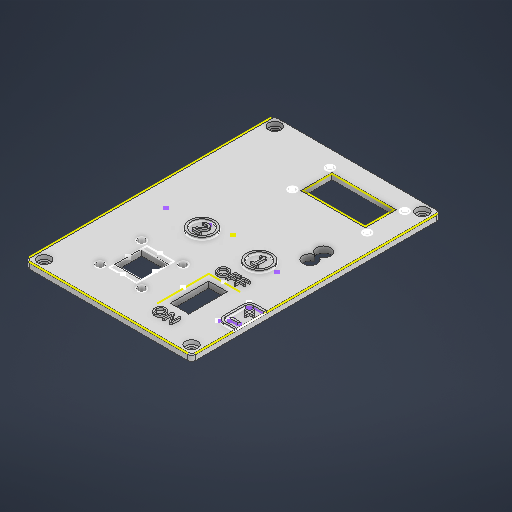
# Autodesk Inventor part: PCB_Housing_06_V4
Saved by Autodesk Inventor 2026.2 (Build 302298010, 298A)
## iProperties
Created: 2026-03-17
Part Number: PCB_Housing_06_V4
Material: Generic
Document SubType Name: Modeling
Designer: vckot
Density: 1 g/cm^3
Appearance: Default
Author: vckot
Autodesk Inventor part; units mm, degrees
ref_plane "YZ Plane" through (0, 0, 0) normal (1, 0, 0) x (0, 1, 0)
ref_plane "XZ Plane" through (0, 0, 0) normal (0, 1, 0) x (-1, 0, 0)
ref_plane "XY Plane" through (0, 0, 0) normal (0, 0, 1) x (1, 0, 0)
sketch "Sketch1" plane through (0, 0, 0) normal (0, 1, 0) x (-1, 0, 0)
  line L0 (-40, 60) -> (40, 60)
  line L1 (40, 60) -> (40, -60)
  line L2 (40, -60) -> (-40, -60)
  line L3 (-40, -60) -> (-40, 60)
  line L4 (-40, 60) -> (40, -60) construction
  line L5 (40, 60) -> (-40, -60) construction
  point P0 (0, 0)
  dimension "d0" = 120
  dimension "d1" = 80
  constraints: 12 end point, 2 midpoint, 2 parallel, 1 horizontal, 1 perpendicular
  measures "d0" distance of L0.end L1.end
  measures "d1" distance of L0.start L0.end
extrude "Extrusion1" add sketch "Sketch1" along normal blind 3
sketch "Sketch2" plane through (0, 3, 0) normal (0, 1, 0) x (1, 0, 0)
  circle A0 centre (35.5, 55.5) radius 2.25
  circle A1 centre (-35.5, -55.5) radius 2.25
  arc A2 (37.5, -54.469224) -> (34.469224, -57.5) centre (35.5, -55.5) ccw
  circle A3 centre (-35.5, 55.5) radius 2.25
  circle A4 centre (35.5, -55.5) radius 2.25
  point P0 (0, 0)
  constraints: 2 centre point, 2 horizontal alignment, 2 vertical alignment
hole "Hole1" at (35.5, 3, -55.5) at (-35.5, 3, 55.5) at (35.5, 3, 55.5) at (-35.5, 3, -55.5) direction (0, -1, 0) diameter 3.75 depth 8 tip angle 118 counterbore diameter 6 counterbore depth 2
sketch "Sketch3" plane through (0, 3, 0) normal (0, 1, 0) x (1, 0, 0)
  line L0 (24.241, -45.543499) -> (24.241, -22.556499)
  line L1 (10.779, -45.543499) -> (24.241, -45.543499)
  line L2 (10.779, -22.556499) -> (10.779, -45.543499)
  line L3 (10.779, -22.556499) -> (24.241, -22.556499)
  arc A0 (26.856832, 17.449996) -> (30.143167, 17.449996) centre (28.499999, 14.999996) ccw
  arc A1 (26.856832, 10.949996) -> (30.143167, 10.949996) centre (28.499999, 8.499996) ccw
  circle A2 centre (28.499999, 8.499996) radius 2.95
  circle A3 centre (28.499999, 14.999996) radius 2.95
  line L4 (28, 35.5) -> (-2, 35.5)
  line L5 (-2, 35.5) -> (-2, 49.5)
  line L6 (-2, 49.5) -> (28, 49.5)
  line L7 (28, 49.5) -> (28, 35.5)
  circle A4 centre (-7, 34) radius 1.1
  circle A5 centre (30, 34) radius 1.1
  circle A6 centre (30, 52) radius 1.1
  circle A7 centre (-7, 52) radius 1.1
  line L8 (31.5, 32.5) -> (31.5, 53.5)
  line L9 (31.5, 53.5) -> (-8.5, 53.5)
  line L10 (-8.5, 53.5) -> (-8.5, 32.5)
  line L11 (-8.5, 32.5) -> (31.5, 32.5)
  line L12 (24.241, -22.556499) -> (10.779, -22.556499)
  line L13 (10.779, -22.556499) -> (10.779, -45.543499)
  line L14 (10.779, -45.543499) -> (24.241, -45.543499)
  line L15 (24.241, -45.543499) -> (24.241, -22.556499)
  arc A8 (12.1379, -23.305799) -> (11.7569, -23.686799) centre (12.1379, -23.686799) ccw
  line L16 (11.7569, -23.686799) -> (11.7569, -23.153399)
  line L17 (11.7569, -23.153399) -> (23.2631, -23.153399)
  line L18 (23.2631, -23.153399) -> (23.2631, -23.686799)
  arc A9 (23.2631, -23.686799) -> (22.8821, -23.305799) centre (22.8821, -23.686799) ccw
  line L19 (22.8821, -23.305799) -> (20.05, -23.305799)
  line L20 (20.05, -23.305799) -> (20.05, -23.559799)
  line L21 (20.05, -23.559799) -> (14.97, -23.559799)
  line L22 (14.97, -23.559799) -> (14.97, -23.305799)
  line L23 (14.97, -23.305799) -> (12.1379, -23.305799)
  line L24 (18.790769, -42.147052) -> (18.797824, -42.147052)
  line L25 (18.797824, -42.147052) -> (19.407999, -41.186537)
  line L26 (19.407999, -41.186537) -> (20.174294, -41.186537)
  line L27 (20.174294, -41.186537) -> (19.317111, -42.295346)
  line L28 (19.317111, -42.295346) -> (19.71607, -43.707864)
  line L29 (19.71607, -43.707864) -> (18.921553, -43.707864)
  line L30 (18.921553, -43.707864) -> (18.739263, -42.870885)
  line L31 (18.739263, -42.870885) -> (18.595587, -43.065169)
  line L32 (18.595587, -43.065169) -> (18.458966, -43.707864)
  line L33 (18.458966, -43.707864) -> (17.828648, -43.707864)
  line L34 (17.828648, -43.707735) -> (17.358303, -43.707735)
  line L35 (17.358303, -43.707735) -> (17.312378, -43.618194)
  spline S0 degree 3 poles (17.312378, -43.618194) (17.183262, -43.69882) (17.011235, -43.7391) (16.883594, -43.7391) knots 0 0 0 0 1 1 1 1
  spline S1 degree 3 poles (16.883594, -43.7391) (16.666279, -43.7391) (16.455181, -43.56555) (16.493385, -43.215144) (16.643637, -42.986824) (16.809283, -42.872511) (16.900399, -42.827654) knots 0.00500991 0.00500991 0.00500991 0.00500991 0.25104614 0.49708236 0.74311859 0.98915482 0.98915482 0.98915482 0.98915482
  spline S2 degree 3 poles (16.900399, -42.827654) (16.834462, -42.726888) (16.785779, -42.608163) (16.814322, -42.473787) knots 0 0 0 0 1 1 1 1
  spline S3 degree 3 poles (16.814322, -42.473787) (16.865314, -42.234156) (17.088333, -42.0908) (17.343615, -42.0908) knots 0 0 0 0 1 1 1 1
  spline S4 degree 3 poles (17.343615, -42.0908) (17.467218, -42.0908) (17.681137, -42.129323) (17.798163, -42.294936) (17.752062, -42.538795) (17.638072, -42.718098) (17.498782, -42.813553) (17.399546, -42.881404) knots 0.00821535 0.00821535 0.00821535 0.00821535 0.2540357 0.49985605 0.62276622 0.74567639 0.99149674 0.99149674 0.99149674 0.99149674
  line L36 (17.399546, -42.881404) -> (17.51019, -43.09865)
  spline S5 degree 3 poles (17.51019, -43.09865) (17.548931, -43.042655) (17.587672, -42.98666) (17.601014, -42.92393) knots 0 0 0 0 1 1 1 1
  line L37 (17.601014, -42.92393) -> (17.91933, -42.92393)
  line L38 (17.91933, -42.92393) -> (18.288607, -41.186537)
  line L39 (18.288607, -41.186537) -> (18.994866, -41.186537)
  line L40 (18.994866, -41.186537) -> (18.790769, -42.147052)
  line L41 (16.779109, -42.103629) -> (16.094081, -42.103629)
  line L42 (16.094081, -42.103629) -> (16.137569, -41.898762)
  spline S6 degree 3 poles (16.137569, -41.898762) (16.160852, -41.789337) (16.203698, -41.588062) (16.058867, -41.588062) knots 0 0 0 0 1 1 1 1
  spline S7 degree 3 poles (16.058867, -41.588062) (15.875231, -41.588062) (15.841172, -41.715125) (15.688773, -42.432031) knots 0 0 0 0 1 1 1 1
  spline S8 degree 3 poles (15.688773, -42.432031) (15.531947, -43.17004) (15.527073, -43.275937) (15.700062, -43.275937) knots 0 0 0 0 1 1 1 1
  spline S9 degree 3 poles (15.700062, -43.275937) (15.813078, -43.275937) (15.883056, -43.162984) (15.949827, -42.848693) knots 0 0 0 0 1 1 1 1
  line L43 (15.949827, -42.848693) -> (15.99107, -42.654473)
  line L44 (15.99107, -42.654473) -> (16.676162, -42.654473)
  line L45 (16.676162, -42.654473) -> (16.642424, -42.813415)
  spline S10 degree 3 poles (16.642424, -42.813415) (16.517028, -43.403065) (16.20838, -43.742115) (15.590444, -43.742115) knots 0.00895212 0.00895212 0.00895212 0.00895212 0.99175551 0.99175551 0.99175551 0.99175551
  spline S11 degree 3 poles (15.590444, -43.742115) (15.27401, -43.742115) (14.887863, -43.619986) (14.820678, -43.200507) (14.894815, -42.739756) (15.015532, -42.174372) (15.128196, -41.693261) (15.356087, -41.359939) (15.610614, -41.189827) (15.990864, -41.109001) (16.642583, -41.140034) (16.885652, -41.421424) (16.852223, -41.758005) (16.818145, -41.919923) knots 0.00651356 0.00651356 0.00651356 0.00651356 0.12992302 0.25333248 0.31503721 0.37674194 0.5001514 0.56185613 0.62356086 0.68526559 0.74697032 0.87037978 0.98786975 0.98786975 0.98786975 0.98786975
  line L46 (16.818171, -41.919928) -> (16.779109, -42.103629)
  line L47 (14.5255, -39.993599) -> (14.5255, -28.106399)
  line L48 (14.5255, -28.106399) -> (20.4945, -28.106399)
  line L49 (20.4945, -28.106399) -> (20.4945, -39.993599)
  line L50 (20.4945, -39.993599) -> (14.5255, -39.993599)
  arc A10 (22.8821, -44.794199) -> (23.2631, -44.413199) centre (22.8821, -44.413199) ccw
  line L51 (23.2631, -44.413199) -> (23.2631, -44.946599)
  line L52 (23.2631, -44.946599) -> (11.7569, -44.946599)
  line L53 (11.7569, -44.946599) -> (11.7569, -44.413199)
  arc A11 (11.7569, -44.413199) -> (12.1379, -44.794199) centre (12.1379, -44.413199) ccw
  line L54 (12.1379, -44.794199) -> (22.8821, -44.794199)
  point P0 (0, 0)
  point P1 (26.856832, 10.949996)
extrude "Extrusion2" cut sketch "Sketch3" against normal through all contours L1 L2 L3 L0 | A3 A0 | A2 A1 | L4 L5 L6 L7 | A8 L16 L17 L18 A9 L19 L20 L21 L22 L23 | L24 L25 L26 L27 L28 L29 L30 L31 L32 L33 L34 L35 S0 S1 S2 S3 S4 L36 S5 L37 L38 L39 L40 | L41 L42 S6 S7 S8 S9 L43 L44 L45 S10 S11 L46 | L47 L48 L49 L50 | A10 L51 L52 L53 A11 L54
sketch "Sketch5" plane through (0, 3, 0) normal (0, 1, 0) x (1, 0, 0)
  circle A0 centre (-5, 33.5) radius 1.75
  circle A1 centre (-5, 51.5) radius 1.75
  circle A2 centre (31, 51.5) radius 1.75
  circle A3 centre (31, 33.5) radius 1.75
  line L0 (28, 35.5) -> (-2, 35.5) projected
  line L1 (-2, 35.5) -> (-2, 49.5) projected
  line L2 (-2, 49.5) -> (28, 49.5) projected
  line L3 (28, 49.5) -> (28, 35.5) projected
  point P0 (0, 0)
  dimension "d27" = 3.5
  dimension "d28" = 2
  dimension "d29" = 3
  dimension "d30" = 2
  dimension "d31" = 3
  dimension "d32" = 3
  dimension "d33" = 3
  dimension "d34" = 2
  dimension "d35" = 2
  constraints: 4 centre point, 3 equal radius
  measures "d27" diameter of A0
  measures "d28" distance from line of A0.centre L0
  measures "d29" distance from line of L1 A0.centre
  measures "d30" distance from line of L2 A1.centre
  measures "d31" distance from line of L1 A1.centre
  measures "d32" distance from line of L3 A2.centre
  measures "d33" distance from line of L3 A3.centre
  measures "d34" distance from line of L0 A3.centre
  measures "d35" distance from line of L2 A2.centre
thicken "Thicken1" operation add thickness 0.5 both sides no extend neighbours yes toward (0, 0, -1) faces at (18, 2, -49.5) (-2, 2, -44.833333) (28, 2, -40.166667) (8, 2, -35.5)
thicken "Thicken2" operation add thickness 0.5 both sides no extend neighbours yes toward (0.6830158, 0, -0.7304036) faces at (30.514896, 2, -17.154687)
thicken "Thicken3" operation add thickness 0.5 both sides no extend neighbours yes toward (0.6830158, 0, -0.7304036) faces at (30.514896, 2, -10.654687)
thicken "Thicken4" operation add thickness 0.75 both sides no extend neighbours yes toward (1, 0, 0) faces at (24.241, 2, 37.881166) (15.266333, 1, 22.556499) (10.779, 2, 30.218832) (15.266333, 2, 45.543499)
sketch "Sketch4" plane through (0, 3, 0) normal (0, 1, 0) x (1, 0, 0)
  line L0 (7.168033, -20.561799) -> (27.698693, -20.561798) construction
  line L1 (27.698693, -20.561798) -> (27.698693, -47.5382) construction
  line L2 (27.698693, -47.5382) -> (7.168033, -47.5382) construction
  line L3 (7.168033, -47.5382) -> (7.168033, -20.561799) construction
  line L4 (10.029, -21.806499) -> (24.991, -21.806499)
  line L5 (10.029, -46.293499) -> (10.029, -21.806499)
  spline S0 degree 2 poles (13.32574, -20.740761) (12.567892, -20.740761) (11.464753, -20.090537) (10.854888, -18.94704) (10.841435, -18.207129) knots 0 0 0 1 2 3 3 3
  spline S1 degree 2 poles (10.841435, -18.207129) (10.854888, -17.467219) (11.460269, -16.323721) (12.567892, -15.673497) (13.32574, -15.673497) knots 0 0 0 1 2 3 3 3
  spline S2 degree 2 poles (13.32574, -15.673497) (14.079103, -15.673497) (15.182242, -16.323721) (15.792107, -17.467219) (15.80556, -18.207129) knots 0 0 0 1 2 3 3 3
  spline S3 degree 2 poles (15.80556, -18.207129) (15.792107, -18.947039) (15.182242, -20.090537) (14.079103, -20.740761) (13.32574, -20.740761) knots 0 0 0 1 2 3 3 3
  spline S4 degree 2 poles (13.32574, -20.018788) (13.872825, -20.018788) (14.635157, -19.538968) (15.038744, -18.71834) (15.038744, -18.207129) knots 0 0 0 1 2 3 3 3
  spline S5 degree 2 poles (15.038744, -18.207129) (15.038744, -17.695918) (14.635157, -16.875291) (13.872825, -16.39547) (13.32574, -16.39547) knots 0 0 0 1 2 3 3 3
  spline S6 degree 2 poles (13.32574, -16.39547) (12.77417, -16.39547) (12.011838, -16.875291) (11.612735, -17.691434) (11.612735, -18.207129) knots 0 0 0 1 2 3 3 3
  spline S7 degree 2 poles (11.612735, -18.207129) (11.612735, -18.722824) (12.011838, -19.538968) (12.77417, -20.018788) (13.32574, -20.018788) knots 0 0 0 1 2 3 3 3
  spline S8 degree 2 poles (17.088072, -20.709371) (16.926637, -20.709371) (16.71139, -20.48964) (16.71139, -20.328205) knots 0 0 0 1 2 2 2
  line L6 (16.71139, -20.328205) -> (16.71139, -16.126412)
  spline S9 degree 2 poles (16.71139, -16.126412) (16.71139, -15.969461) (16.926637, -15.740761) (17.088071, -15.740761) knots 0 0 0 1 2 2 2
  line L7 (17.088071, -15.740761) -> (19.760717, -15.740761)
  spline S10 degree 2 poles (19.760717, -15.740761) (19.913184, -15.740761) (20.12843, -15.956008) (20.12843, -16.10399) knots 0 0 0 1 2 2 2
  spline S11 degree 2 poles (20.12843, -16.10399) (20.12843, -16.260941) (19.913184, -16.462734) (19.760717, -16.462734) knots 0 0 0 1 2 2 2
  line L8 (19.760717, -16.462734) -> (17.478206, -16.462734)
  line L9 (17.478206, -16.462734) -> (17.478206, -17.8439)
  line L10 (17.478206, -17.8439) -> (19.518565, -17.8439)
  spline S12 degree 2 poles (19.518565, -17.8439) (19.675515, -17.8439) (19.886278, -18.054663) (19.886278, -18.207129) knots 0 0 0 1 2 2 2
  spline S13 degree 2 poles (19.886278, -18.207129) (19.886278, -18.359595) (19.675516, -18.565873) (19.518565, -18.565873) knots 0 0 0 1 2 2 2
  line L11 (19.518565, -18.565873) -> (17.478206, -18.565873)
  line L12 (17.478206, -18.565873) -> (17.478206, -20.328205)
  spline S14 degree 2 poles (17.478206, -20.328205) (17.478206, -20.48964) (17.249507, -20.709371) (17.088072, -20.709371) knots 0 0 0 1 2 2 2
  spline S15 degree 2 poles (21.267444, -20.709371) (21.106009, -20.709371) (20.890762, -20.48964) (20.890762, -20.328205) knots 0 0 0 1 2 2 2
  line L13 (20.890762, -20.328205) -> (20.890762, -16.126411)
  spline S16 degree 2 poles (20.890762, -16.126411) (20.890762, -15.969461) (21.106009, -15.740761) (21.267444, -15.740761) knots 0 0 0 1 2 2 2
  line L14 (21.267444, -15.740761) -> (23.940089, -15.740761)
  spline S17 degree 2 poles (23.940089, -15.740761) (24.092556, -15.740761) (24.307802, -15.956008) (24.307802, -16.10399) knots 0 0 0 1 2 2 2
  spline S18 degree 2 poles (24.307802, -16.10399) (24.307802, -16.260941) (24.092556, -16.462734) (23.940089, -16.462734) knots 0 0 0 1 2 2 2
  line L15 (23.940089, -16.462734) -> (21.657578, -16.462734)
  line L16 (21.657578, -16.462734) -> (21.657578, -17.8439)
  line L17 (21.657578, -17.8439) -> (23.697937, -17.8439)
  spline S19 degree 2 poles (23.697937, -17.8439) (23.854888, -17.8439) (24.06565, -18.054663) (24.06565, -18.207129) knots 0 0 0 1 2 2 2
  spline S20 degree 2 poles (24.06565, -18.207129) (24.06565, -18.359595) (23.854888, -18.565873) (23.697937, -18.565873) knots 0 0 0 1 2 2 2
  line L18 (23.697937, -18.565873) -> (21.657578, -18.565873)
  line L19 (21.657578, -18.565873) -> (21.657578, -20.328205)
  spline S21 degree 2 poles (21.657578, -20.328205) (21.657578, -20.48964) (21.428879, -20.709371) (21.267444, -20.709371) knots 0 0 0 1 2 2 2
  spline S22 degree 2 poles (14.747265, -52.426502) (13.989418, -52.426502) (12.886279, -51.776278) (12.276413, -50.63278) (12.26296, -49.89287) knots 0 0 0 1 2 3 3 3
  spline S23 degree 2 poles (12.26296, -49.89287) (12.276413, -49.152959) (12.881794, -48.009461) (13.989418, -47.359237) (14.747265, -47.359237) knots 0 0 0 1 2 3 3 3
  spline S24 degree 2 poles (14.747265, -47.359237) (15.500628, -47.359237) (16.603767, -48.009461) (17.213633, -49.152959) (17.227086, -49.892869) knots 0 0 0 1 2 3 3 3
  spline S25 degree 2 poles (17.227086, -49.892869) (17.213633, -50.63278) (16.603768, -51.776277) (15.500629, -52.426502) (14.747265, -52.426502) knots 0 0 0 1 2 3 3 3
  spline S26 degree 2 poles (14.747265, -51.704529) (15.29435, -51.704529) (16.056682, -51.224708) (16.46027, -50.40408) (16.46027, -49.892869) knots 0 0 0 1 2 3 3 3
  spline S27 degree 2 poles (16.46027, -49.892869) (16.46027, -49.381659) (16.056682, -48.561031) (15.29435, -48.08121) (14.747265, -48.08121) knots 0 0 0 1 2 3 3 3
  spline S28 degree 2 poles (14.747265, -48.08121) (14.195696, -48.08121) (13.433364, -48.561031) (13.034261, -49.377174) (13.034261, -49.892869) knots 0 0 0 1 2 3 3 3
  spline S29 degree 2 poles (13.034261, -49.892869) (13.034261, -50.408565) (13.433364, -51.224708) (14.195696, -51.704529) (14.747265, -51.704529) knots 0 0 0 1 2 3 3 3
  spline S30 degree 2 poles (18.509597, -52.395112) (18.348162, -52.395112) (18.132916, -52.175381) (18.132916, -52.013946) knots 0 0 0 1 2 2 2
  line L20 (18.132916, -52.013946) -> (18.132915, -47.915291)
  spline S31 degree 2 poles (18.132915, -47.915291) (18.132915, -47.704529) (18.433364, -47.395112) (18.64861, -47.395112) knots 0 0 0 1 2 2 2
  line L21 (18.64861, -47.395112) -> (18.738297, -47.395112)
  spline S32 degree 2 poles (18.738297, -47.395112) (18.872826, -47.395112) (19.097041, -47.520672) (19.150853, -47.596905) knots 0 0 0 1 2 2 2
  line L22 (19.150853, -47.596905) -> (21.688969, -51.413049)
  line L23 (21.688969, -51.413049) -> (21.688969, -47.776277)
  spline S33 degree 2 poles (21.688969, -47.776277) (21.688969, -47.619327) (21.904216, -47.395111) (22.065651, -47.395111) knots 0 0 0 1 2 2 2
  spline S34 degree 2 poles (22.065651, -47.395111) (22.227086, -47.395111) (22.455785, -47.619327) (22.455785, -47.776277) knots 0 0 0 1 2 2 2
  line L24 (22.455785, -47.776277) -> (22.455785, -51.874932)
  spline S35 degree 2 poles (22.455785, -51.874932) (22.455785, -52.090179) (22.146368, -52.395111) (21.931122, -52.395111) knots 0 0 0 1 2 2 2
  line L25 (21.931122, -52.395111) -> (21.84592, -52.395111)
  spline S36 degree 2 poles (21.84592, -52.395111) (21.715875, -52.395111) (21.496144, -52.274035) (21.433364, -52.188833) knots 0 0 0 1 2 2 2
  line L26 (21.433364, -52.188833) -> (18.899732, -48.368206)
  line L27 (18.899732, -48.368206) -> (18.899732, -52.013946)
  spline S37 degree 2 poles (18.899732, -52.013946) (18.899732, -52.175381) (18.671032, -52.395112) (18.509597, -52.395112) knots 0 0 0 1 2 2 2
  point P0 (0, 0)
  point P1 (27.698693, -34.049999)
  point P2 (10.029, -34.049999)
  constraints: 2 midpoint, 1 horizontal alignment, 2 other
extrude "Extrusion3" add sketch "Sketch4" along normal blind 1
fillet "Fillet1" radius 2 4 edges at (-40, 1.5, -60) (-40, 1.5, 60) (40, 1.5, -60) (40, 1.5, 60)
fillet "Fillet2" radius 0.5 8 edges at (39.4142, 3, -59.4142) (0, 3, -60) (-39.4142, 3, -59.4142) (-40, 3, 0) (-39.4142, 3, 59.4142) (0, 3, 60) (39.4142, 3, 59.4142) (40, 3, 0)
sketch "Sketch6" plane through (0, 3, 0) normal (0, 1, 0) x (1, 0, 0)
  line L0 (8.988356, -6.885061) -> (26.031643, -6.885061) construction
  line L1 (26.031643, -6.885061) -> (26.031643, -3.114939) construction
  line L2 (26.031643, -3.114939) -> (8.988356, -3.114939) construction
  line L3 (8.988356, -3.114939) -> (8.988356, -6.885061) construction
  circle A0 centre (17.51, -5) radius 5
  circle A1 centre (17.51, -5) radius 6
  line L4 (10.029, -21.806499) -> (24.991, -21.806499)
  line L5 (-16.5, -25.049999) -> (-3.5, -25.049999)
  line L6 (-3.5, -25.049999) -> (-3.5, -43.049999)
  line L7 (-3.5, -43.049999) -> (-16.5, -43.049999)
  line L8 (-16.5, -43.049999) -> (-16.5, -25.049999)
  line L9 (-40, 58) -> (-40, -58)
  line L10 (-38, -60) -> (38, -60)
  line L11 (-16.5, -27.549999) -> (-3.5, -27.549999)
  line L12 (-3.5, -27.549999) -> (-3.5, -40.549999)
  line L13 (-3.5, -40.549999) -> (-16.5, -40.549999)
  line L14 (-16.5, -40.549999) -> (-16.5, -27.549999)
  circle A2 centre (-10, -5) radius 5
  circle A3 centre (-10, -5) radius 6
  line L15 (-27.288736, -1.885737) -> (7.288736, -1.885737) construction
  line L16 (7.288736, -1.885737) -> (7.288736, -8.114263) construction
  line L17 (7.288736, -8.114263) -> (-27.288736, -8.114263) construction
  line L18 (-27.288736, -8.114263) -> (-27.288736, -1.885737) construction
  circle A4 centre (0, -24.049999) radius 1.875
  circle A5 centre (-20, -24.049999) radius 1.875
  circle A6 centre (-20, -44.049999) radius 1.875
  circle A7 centre (0, -44.049999) radius 1.875
  line L19 (10.029, -46.293499) -> (10.029, -21.806499)
  line L20 (33.93144, -26.461168) -> (37.900698, -26.461168) construction
  line L21 (37.900698, -26.461168) -> (37.900698, -29.874369) construction
  line L22 (37.900698, -29.874369) -> (33.93144, -29.874369) construction
  line L23 (33.93144, -29.874369) -> (33.93144, -26.461168) construction
  line L24 (40, -58) -> (40, 58)
  line L25 (40, -39.53) -> (35, -39.53)
  line L26 (32, -36.53) -> (32, -27.18)
  line L27 (35, -24.18) -> (40, -24.18)
  line L28 (40, -24.18) -> (40, -39.53)
  arc A8 (35, -24.18) -> (32, -27.18) centre (35, -27.18) ccw
  arc A9 (32, -36.53) -> (35, -39.53) centre (35, -36.53) ccw
  line L29 (34.892818, -35.202032) -> (38.482019, -35.202032)
  line L30 (38.982019, -35.702032) -> (38.982019, -35.702032)
  line L31 (38.482019, -36.202032) -> (34.892818, -36.202032)
  line L32 (34.392818, -35.702032) -> (34.392818, -35.702032)
  arc A10 (34.892818, -35.202032) -> (34.392818, -35.702032) centre (34.892818, -35.702032) ccw
  arc A11 (34.392818, -35.702032) -> (34.892818, -36.202032) centre (34.892818, -35.702032) ccw
  arc A12 (38.482019, -36.202032) -> (38.982019, -35.702032) centre (38.482019, -35.702032) ccw
  arc A13 (38.982019, -35.702032) -> (38.482019, -35.202032) centre (38.482019, -35.702032) ccw
  line L33 (40, -38.65132) -> (35, -38.65132)
  line L34 (33, -36.65132) -> (33, -27.30132)
  line L35 (35, -25.30132) -> (40, -25.30132)
  line L36 (40, -25.30132) -> (40, -38.65132)
  arc A14 (35, -25.30132) -> (33, -27.30132) centre (35, -27.30132) ccw
  arc A15 (33, -36.65132) -> (35, -38.65132) centre (35, -36.65132) ccw
  spline S0 degree 2 poles (-11.528251, -8) (-11.75426, -8) (-12.050224, -7.714798) (-12.050224, -7.483408) knots 0 0 0 1 2 2 2
  spline S1 degree 2 poles (-12.050224, -7.483408) (-12.050224, -7.026009) (-11.555157, -6.29417) (-10.78565, -5.696861) (-9.935426, -5.164126) (-9.208969, -4.658296) (-8.756951, -4.120179) (-8.756951, -3.813453) knots 0 0 0 1 2 3 4 5 6 6 6
  spline S2 degree 2 poles (-8.756951, -3.813453) (-8.756951, -3.409865) (-9.295067, -2.87713) (-9.973094, -2.87713) knots 0 0 0 1 2 2 2
  spline S3 degree 2 poles (-9.973094, -2.87713) (-10.376682, -2.87713) (-11.076233, -3.043946) (-11.329148, -3.156951) knots 0 0 0 1 2 2 2
  spline S4 degree 2 poles (-11.329148, -3.156951) (-11.345292, -3.167713) (-11.47444, -3.210762) (-11.539014, -3.210762) knots 0 0 0 1 2 2 2
  spline S5 degree 2 poles (-11.539014, -3.210762) (-11.711211, -3.210762) (-11.93722, -2.973991) (-11.93722, -2.807175) knots 0 0 0 1 2 2 2
  spline S6 degree 2 poles (-11.93722, -2.807175) (-11.93722, -2.55426) (-11.711211, -2.430493) knots 0 0 0 1 1 1
  spline S7 degree 2 poles (-11.711211, -2.430493) (-11.361435, -2.252915) (-10.419731, -2) (-9.838565, -2) knots 0 0 0 1 2 2 2
  spline S8 degree 2 poles (-9.838565, -2) (-9.295067, -2) (-8.396413, -2.441256) (-7.858296, -3.226906) (-7.858296, -3.75426) knots 0 0 0 1 2 3 3 3
  spline S9 degree 2 poles (-7.858296, -3.75426) (-7.858296, -4.195516) (-8.288789, -4.943498) (-8.972197, -5.562332) (-9.741704, -6.095067) (-10.484305, -6.56861) (-11.033184, -7.03139) (-11.130045, -7.133632) knots 0 0 0 1 2 3 4 5 6 6 6
  line L37 (-11.130045, -7.133632) -> (-8.347982, -7.133632)
  spline S10 degree 2 poles (-8.347982, -7.133632) (-8.165022, -7.133632) (-7.912108, -7.386547) (-7.912108, -7.569507) knots 0 0 0 1 2 2 2
  spline S11 degree 2 poles (-7.912108, -7.569507) (-7.912108, -7.752466) (-8.165022, -8) (-8.347982, -8) knots 0 0 0 1 2 2 2
  line L38 (-8.347982, -8) -> (-11.528251, -8)
  spline S12 degree 2 poles (16.466053, -7.959641) (16.277713, -7.959641) (16.03556, -7.712108) (16.03556, -7.529148) knots 0 0 0 1 2 2 2
  spline S13 degree 2 poles (16.03556, -7.529148) (16.03556, -7.346188) (16.277713, -7.093273) (16.466053, -7.093273) knots 0 0 0 1 2 2 2
  line L39 (16.466053, -7.093273) -> (17.359327, -7.093273)
  line L40 (17.359327, -7.093273) -> (17.359327, -3.084305)
  line L41 (17.359327, -3.084305) -> (16.643632, -3.487892)
  spline S14 degree 2 poles (16.643632, -3.487892) (16.595201, -3.504036) (16.49834, -3.541704) (16.417623, -3.541704) knots 0 0 0 1 2 2 2
  spline S15 degree 2 poles (16.417623, -3.541704) (16.223901, -3.541704) (15.976367, -3.299551) (15.976367, -3.105829) knots 0 0 0 1 2 2 2
  spline S16 degree 2 poles (15.976367, -3.105829) (15.976367, -2.826009) (16.261569, -2.680717) knots 0 0 0 1 1 1
  line L42 (16.261569, -2.680717) -> (17.386233, -2.09417)
  spline S17 degree 2 poles (17.386233, -2.09417) (17.488475, -2.040358) (17.628385, -2.040358) knots 0 0 0 1 1 1
  line L43 (17.628385, -2.040358) -> (17.800583, -2.040358)
  spline S18 degree 2 poles (17.800583, -2.040358) (17.999686, -2.040358) (18.284888, -2.320179) (18.284888, -2.519282) knots 0 0 0 1 2 2 2
  line L44 (18.284888, -2.519282) -> (18.284888, -7.093273)
  line L45 (18.284888, -7.093273) -> (19.011345, -7.093273)
  spline S19 degree 2 poles (19.011345, -7.093273) (19.194305, -7.093273) (19.452601, -7.346188) (19.452601, -7.529148) knots 0 0 0 1 2 2 2
  spline S20 degree 2 poles (19.452601, -7.529148) (19.452601, -7.712108) (19.194305, -7.959641) (19.011345, -7.959641) knots 0 0 0 1 2 2 2
  line L46 (19.011345, -7.959641) -> (16.466053, -7.959641)
  spline S21 degree 2 poles (36.73144, -31.301527) (36.536821, -31.301527) (36.260588, -31.025294) (36.260588, -30.824397) knots 0 0 0 1 2 2 2
  line L47 (36.260588, -30.824397) -> (36.260588, -29.349061)
  line L48 (36.260588, -29.349061) -> (34.778973, -29.349061)
  spline S22 degree 2 poles (34.778973, -29.349061) (34.584354, -29.349061) (34.314399, -29.079106) (34.314399, -28.884487) knots 0 0 0 1 2 2 2
  spline S23 degree 2 poles (34.314399, -28.884487) (34.314399, -28.68359) (34.584354, -28.413635) (34.778973, -28.413635) knots 0 0 0 1 2 2 2
  line L49 (34.778973, -28.413635) -> (36.260588, -28.413635)
  line L50 (36.260588, -28.413635) -> (36.260588, -26.932021)
  spline S24 degree 2 poles (36.260588, -26.932021) (36.260588, -26.731124) (36.536821, -26.461169) (36.73144, -26.461169) knots 0 0 0 1 2 2 2
  spline S25 degree 2 poles (36.73144, -26.461169) (36.938615, -26.461169) (37.20857, -26.731124) (37.20857, -26.932021) knots 0 0 0 1 2 2 2
  line L51 (37.20857, -26.932021) -> (37.20857, -28.413635)
  line L52 (37.20857, -28.413635) -> (38.67135, -28.413635)
  spline S26 degree 2 poles (38.67135, -28.413635) (38.878525, -28.413635) (39.14848, -28.68359) (39.14848, -28.884487) knots 0 0 0 1 2 2 2
  spline S27 degree 2 poles (39.14848, -28.884487) (39.14848, -29.079106) (38.878525, -29.349061) (38.67135, -29.349061) knots 0 0 0 1 2 2 2
  line L53 (38.67135, -29.349061) -> (37.20857, -29.349061)
  line L54 (37.20857, -29.349061) -> (37.20857, -30.824397)
  spline S28 degree 2 poles (37.20857, -30.824397) (37.20857, -31.019016) (36.938615, -31.301527) (36.73144, -31.301527) knots 0 0 0 1 2 2 2
  point P0 (0, 0)
  point P1 (17.51, -21.806499)
  point P2 (-10, -43.049999)
  point P3 (-3.5, -34.049999)
  point P4 (-16.5, -34.049999)
  point P5 (-16.5, -34.049999)
  point P6 (-10, -25.049999)
  point P7 (-10, -1.885737)
  point P8 (-27.288736, -5)
  point P9 (26.031643, -5)
  point P10 (17.51, -6.885061)
  point P11 (-16.5, -40.549999)
  point P12 (-3.5, -27.549999)
  point P13 (-3.5, -34.049999)
  point P14 (10.029, -34.049999)
  point P15 (32, -24.18)
  point P16 (32, -39.53)
  point P17 (33, -25.30132)
  point P18 (33, -38.65132)
  dimension "d38" = 12
  dimension "d39" = 10
  dimension "d40" = 18
  dimension "d41" = 13
  dimension "d42" = 30
  dimension "d44" = 13
  dimension "d45" = 55
  dimension "d46" = 12
  dimension "d47" = 10
  dimension "d48" = 3.75
  dimension "d50" = 3.5
  dimension "d51" = 3.5
  dimension "d52" = 3.5
  dimension "d53" = 3.5
  dimension "d62" = 8
  dimension "d63" = 15.35
  dimension "d64" = 20.47
  dimension "d65" = 3
  dimension "d66" = 1
  dimension "d67" = 0.5
  dimension "d68" = 7
  dimension "d69" = 13.35
  dimension "d70" = 2
  constraints: 40 end point, 16 centre point, 16 point on circle, 16 tangent, 12 midpoint, 12 point on line, 10 parallel, 8 equal radius, 6 horizontal alignment, 6 vertical alignment, 5 horizontal, 5 perpendicular, 3 coincident, 6 other
  measures "d38" diameter of A1
  measures "d39" diameter of A0
  measures "d40" distance between parallel lines of L7 L5
  measures "d41" distance between parallel lines of L8 L6
  measures "d42" distance from line of L9 point (-10, -43.05)
  measures "d44" distance between parallel lines of L13 L11
  measures "d45" distance from line of L10 A1.centre
  measures "d46" diameter of A3
  measures "d47" diameter of A2
  measures "d48" diameter of A4
  measures "d50" distance from line of A4.centre L11
  measures "d51" distance from line of A4.centre L12
  measures "d52" distance from line of L13 A7.centre
  measures "d53" distance from line of A6.centre L8
  measures "d62" distance of point (32, -24.18) L27.end
  measures "d63" distance of point (32, -39.53) point (32, -24.18)
  measures "d64" distance between parallel lines of L10 L25
  measures "d65" radius of A8
  measures "d66" distance between parallel lines of L31 L29
  measures "d67" radius of A10
  measures "d68" distance of point (33, -25.301) L35.end
  measures "d69" distance of point (33, -38.651) point (33, -25.301)
  measures "d70" radius of A14
extrude "Extrusion5" cut sketch "Sketch6" against normal blind 2.5 contours L11 L6 L13 L8
extrude "Extrusion7" cut sketch "Sketch6" against normal blind 10 contours L11 L6 L13 L8 | A4 | A5 | A6 | A7
thicken "Thicken5" operation add thickness 3 both sides no extend neighbours yes toward (-1, 0, 0) faces at (24.991, 2, 38.131166) (20.003666, 2, 21.806499) (10.029, 1, 29.968832) (15.016333, 2, 46.293499)
extrude "Extrusion8" add sketch "Sketch6" along normal blind 1 contours A1 | A3 | L25 A9 L26 A8 L27 L24 L35 A14 L34 A15 L33 | L29 A13 A12 L31 A11 A10 | S0 S1 S2 S3 S4 S5 S6 S7 S8 S9 L37 S10 S11 L38 | S12 S13 L39 L40 L41 S14 S15 S16 L42 S17 L43 S18 L44 L45 S19 S20 L46 | S21 L47 L48 S22 S23 L49 L50 S24 S25 L51 L52 S26 S27 L53 L54 S28
body "Solid1"
